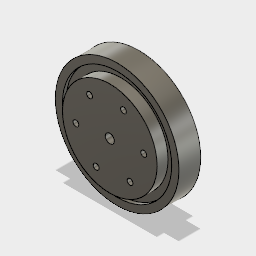
Wheel v3 (Autodesk Fusion 360 design; units mm, degrees)
Autodesk Fusion 360 part; units mm, degrees
sketch "Sketch1" plane through (0, 0, 0) normal (0, 1, 0) x (1, 0, 0)
  line L0 (-63.5, 63.5) -> (63.5, 63.5)
  line L1 (63.5, 63.5) -> (63.5, -63.5)
  line L2 (63.5, -63.5) -> (-63.5, -63.5)
  line L3 (-63.5, -63.5) -> (-63.5, 63.5)
  constraint horizontal L0
  constraint vertical L1
  constraint horizontal L2
  constraint vertical L3
sketch "Sketch6" plane through (0, 0, 0) normal (0, 1, 0) x (1, 0, 0)
  line L0 (-139.6725, 0.0069) -> (-172.6925, 0.0069)
  line L1 (-172.6925, -25.3931) -> (-139.6725, -25.3931)
  line L2 (-139.6725, -25.3931) -> (-139.6725, 0.0069)
  line L3 (-172.6925, -7.6131) -> (-177.7725, -7.6131)
  line L4 (-177.7725, -7.6131) -> (-177.7725, -5.0731)
  line L5 (-177.7725, -5.0731) -> (-182.8525, -5.0731)
  line L6 (-182.8525, -5.0731) -> (-182.8525, -20.3131)
  line L7 (-182.8525, -20.3131) -> (-177.7725, -20.3131)
  line L8 (-177.7725, -20.3131) -> (-177.7725, -17.7731)
  line L9 (-177.7725, -17.7731) -> (-172.6925, -17.7731)
  line L10 (-172.6925, 0.0069) -> (-172.6925, -7.6131)
  line L11 (-172.6925, -17.7731) -> (-172.6925, -25.3931)
  constraint horizontal L0
  constraint vertical L10
  constraint horizontal L1
  constraint vertical L2
  constraint perpendicular L3 L10
  constraint perpendicular L3 L4
  constraint perpendicular L4 L5
  constraint perpendicular L5 L6
  constraint perpendicular L6 L7
  constraint perpendicular L7 L8
  constraint perpendicular L8 L9
  constraint collinear L10 L11
revolve "Revolve2" add sketch "Sketch6" angle 360 about axis through (-139.6725, 0, 25.3931) along (0, 0, -1)
sketch "Sketch7" plane through (0, 0, 25.3931) normal (0, 0, 1) x (1, 0, 0)
  circle A0 centre (-139.6725, 0) radius 33.02
  circle A1 centre (-139.6725, 0) radius 3.175
  dimension "d11" = 6.35
  constraint concentric A0 A1
  measures "d11" diameter of A1
extrude "Extrude4" cut sketch "Sketch7" against normal blind 45.72 contours A1
sketch "Sketch8" plane through (0, 0, 25.3931) normal (0, 0, 1) x (1, 0, 0)
  circle A0 centre (-139.6725, 0) radius 3.175
  circle A1 centre (-139.6725, 0) radius 33.02
  circle A2 centre (-139.6725, 0) radius 23.8125
  dimension "d14" = 47.625
  dimension "d15" = 60
  dimension "d16" = 60
  dimension "d17" = 60
  dimension "d18" = 60
  dimension "d19" = 60
  constraint concentric A0 A2
  constraint coincident A2
  constraint coincident A2 origin
  measures "d14" diameter of A2
  measures "d16" angle of origin
  measures "d19" angle of origin
hole "Hole1" at (-153.8022, 19.1673, 25.3931) at (-130.138, 21.8204, 25.3931) at (-116.0082, 2.6531, 25.3931) at (-125.5427, -19.1673, 25.3931) at (-149.2069, -21.8204, 25.3931) at (-163.3367, -2.6531, 25.3931) direction (0, 0, -1) diameter 4.064 depth 50.8 tip angle 118
